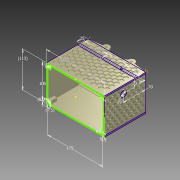
# Autodesk Inventor part: Box2
Saved by Autodesk Inventor 2015 (Build 190159000, 159)
## iProperties
Created: 2015-04-29
Part Number: Box2
Material: Nylon 6/6
Document SubType Name: Modeling
Designer: Akovo_000
Mass: 174.849 g
Surface Area: 2151.16 cm^2
Volume: 154.734 cm^3
Density: 1.13 g/cm^3
Appearance: Nylon 6
Author: Akovo_000
Autodesk Inventor part; units mm, degrees
(part 1 of 2)
ref_plane "YZ Plane" through (0, 0, 0) normal (1, 0, 0) x (0, 1, 0)
ref_plane "XZ Plane" through (0, 0, 0) normal (0, 1, 0) x (-1, 0, 0)
ref_plane "XY Plane" through (0, 0, 0) normal (0, 0, 1) x (1, 0, 0)
sketch "BasicBox" plane through (0, 0, 0) normal (0, 1, 0) x (-1, 0, 0)
  line L0 (88.196, 44.8878) -> (-86.804, 44.8878)
  line L1 (-86.804, 44.8878) -> (-86.804, -60.1122)
  line L2 (-86.804, -60.1122) -> (88.196, -60.1122)
  line L3 (88.196, -60.1122) -> (88.196, 44.8878)
  line L4 (92.196, 48.8878) -> (-90.804, 48.8878)
  line L5 (-90.804, 48.8878) -> (-90.804, -64.1122)
  line L6 (-90.804, -64.1122) -> (92.196, -64.1122)
  line L7 (92.196, -64.1122) -> (92.196, 48.8878)
  line L8 (88.196, 44.8878) -> (88.196, 45.3878) construction
  line L9 (88.196, 44.8878) -> (88.696, 44.8878) construction
  line L10 (88.196, -60.1122) -> (88.196, -60.6122) construction
  line L11 (88.196, -60.1122) -> (88.696, -60.1122) construction
  line L12 (-86.804, -60.1122) -> (-86.804, -60.6122) construction
  line L13 (-86.804, 44.8878) -> (-86.804, 45.3878) construction
  line L14 (-86.804, 44.8878) -> (-87.304, 44.8878) construction
  line L15 (-86.804, -60.1122) -> (-87.304, -60.1122) construction
  line L16 (-87.304, -60.6122) -> (-87.304, -60.1122)
  line L17 (-87.304, 45.3878) -> (-86.804, 45.3878)
  line L18 (88.696, 45.3878) -> (88.696, -60.1122)
  line L19 (88.696, -60.6122) -> (88.196, -60.6122)
  line L20 (88.696, 44.8878) -> (92.196, 44.8878) construction
  line L21 (88.196, 45.3878) -> (88.196, 48.8878) construction
  line L22 (-86.804, 45.3878) -> (88.696, 45.3878)
  line L23 (-87.304, 44.8878) -> (-87.304, 45.3878)
  line L24 (-87.304, -60.1122) -> (-87.304, 44.8878)
  line L25 (-86.804, -60.6122) -> (-87.304, -60.6122)
  line L26 (88.696, -60.1122) -> (88.696, -60.6122)
  line L27 (88.196, -60.6122) -> (-86.804, -60.6122)
  line L28 (88.696, -60.1122) -> (92.196, -60.1122) construction
  line L29 (88.196, -60.6122) -> (88.196, -64.1122) construction
  line L30 (-87.304, 44.8878) -> (-90.804, 44.8878) construction
  line L31 (-86.804, 45.3878) -> (-86.804, 48.8878) construction
  line L32 (-87.304, -60.1122) -> (-90.804, -60.1122) construction
  line L33 (-86.804, -60.6122) -> (-86.804, -64.1122) construction
  line L34 (-76.804, -60.1122) -> (-76.804, -50.1122)
  line L35 (-76.804, -50.1122) -> (-86.804, -50.1122)
  line L36 (-76.804, 44.8878) -> (-76.804, 34.8878)
  line L37 (-76.804, 34.8878) -> (-86.804, 34.8878)
  line L38 (78.696, 44.8878) -> (78.696, 34.8878)
  line L39 (78.696, 34.8878) -> (88.196, 34.8878)
  line L40 (88.696, -50.1122) -> (78.696, -50.1122)
  line L41 (78.696, -50.1122) -> (78.696, -60.1122)
  line L42 (78.696, 44.8878) -> (78.696, 48.8878)
  line L43 (88.196, 34.8878) -> (92.196, 34.8878)
  line L44 (78.696, -60.1122) -> (78.696, -64.1122)
  line L45 (88.696, -50.1122) -> (92.196, -50.1122)
  line L46 (-80.7418, -53.1122) -> (-78.721, -56.6122)
  line L47 (-78.721, -56.6122) -> (-80.7418, -60.1122)
  line L48 (-80.7418, -60.1122) -> (-84.7832, -60.1122)
  line L49 (-84.7832, -60.1122) -> (-86.804, -56.6122)
  line L50 (-86.804, -56.6122) -> (-84.7832, -53.1122)
  line L51 (-84.7832, -53.1122) -> (-80.7418, -53.1122)
  line L52 (-80.7418, 44.8878) -> (-78.721, 41.3878)
  line L53 (-78.721, 41.3878) -> (-80.7418, 37.8878)
  line L54 (-80.7418, 37.8878) -> (-84.7832, 37.8878)
  line L55 (-84.7832, 37.8878) -> (-86.804, 41.3878)
  line L56 (-86.804, 41.3878) -> (-84.7832, 44.8878)
  line L57 (-84.7832, 44.8878) -> (-80.7418, 44.8878)
  line L58 (86.1753, 44.8878) -> (88.196, 41.3878)
  line L59 (88.196, 41.3878) -> (86.1753, 37.8878)
  line L60 (86.1753, 37.8878) -> (82.1339, 37.8878)
  line L61 (82.1339, 37.8878) -> (80.1131, 41.3878)
  line L62 (80.1131, 41.3878) -> (82.1339, 44.8878)
  line L63 (82.1339, 44.8878) -> (86.1753, 44.8878)
  line L64 (86.1753, -53.1122) -> (88.196, -56.6122)
  line L65 (88.196, -56.6122) -> (86.1753, -60.1122)
  line L66 (86.1753, -60.1122) -> (82.1339, -60.1122)
  line L67 (82.1339, -60.1122) -> (80.1131, -56.6122)
  line L68 (80.1131, -56.6122) -> (82.1339, -53.1122)
  line L69 (82.1339, -53.1122) -> (86.1753, -53.1122)
  circle A0 centre (84.1546, 41.3878) radius 2
  circle A1 centre (84.1546, -56.6122) radius 2
  circle A2 centre (-82.7625, -56.6122) radius 2
  circle A3 centre (-82.7625, 41.3878) radius 2
  point P0 (0, 0)
  dimension "d2" = 105
  dimension "d3" = 175
  dimension "d4" = 4
  dimension "d68" = 0.5
  dimension "d71" = 4
  dimension "d94" = 10
  dimension "d95" = 183
  dimension "d96" = 113
  dimension "d97" = 7
  dimension "d98" = 0
  dimension "d101" = 0
  dimension "d102" = 4
  dimension "d105" = 0
  dimension "d106" = 0
  dimension "d109" = 7.5
  dimension "d110" = 8.0414
  constraints: 140 end point, 29 point on line, 22 perpendicular, 14 equal length, 9 parallel, 6 vertical, 5 collinear, 4 centre point, 4 coincident, 4 horizontal, 3 equal radius, 52 other
  measures "d2" distance of L28.end L20.end
  measures "d3" distance of L29.end L33.end
  measures "d4" distance of L6.end L28.end
  measures "d68" distance of L16.start L12.end
  measures "d71" distance of L6.end L29.end
  measures "d94" distance of L34.start L34.end
  measures "d95" distance between parallel lines of L7 L5
  measures "d96" distance between parallel lines of L4 L6
  measures "d97" distance between parallel lines of L51 L48
  measures "d98" distance from line of L1 L49.end
  measures "d101" distance from line of L3 L64.end
  measures "d102" diameter of A0
  measures "d105" distance from line of L1 L55.end
  measures "d106" distance from line of L3 L58.end
  measures "d109" distance from line of L6 point (84.155, -56.612)
  measures "d110" distance from line of L7 point (84.155, -56.612)
extrude "Extrusion1" add sketch "BasicBox" along normal blind 131 contours L0 L42 L22 L18 L43 L3 | L43 L18 L40 L3 | L0 L1 L2 L44 L27 L25 L16 L24 L23 L17 L22 L42 | L40 L18 L26 L19 L27 L44 L2 L3 | L43 L7 L45 L18 | L18 L22 L42 L4 L7 L43 | L22 L17 L23 L24 L16 L25 L27 L44 L6 L5 L4 L42 | L45 L7 L6 L44 L27 L19 L26 L18
sketch "LongerHonycomb" plane through (-92.196, 0, 48.8878) normal (0, 0, 1) x (1, 0, 0)
  line L0 (0, 131) -> (183, 131)
  line L1 (183, 131) -> (183, 0)
  line L2 (183, 0) -> (0, 0)
  line L3 (0, 0) -> (0, 131)
  line L4 (0, 131) -> (183, 131) projected
  line L5 (179, 131) -> (179, 0)
  line L6 (4, 131) -> (4, 0)
  line L7 (179, 131) -> (4, 131) projected
  line L8 (4, 0) -> (179, 0) projected
  line L9 (18.2583, 115) -> (10.7528, 115)
  line L10 (10.7528, 115) -> (7, 121.5)
  line L11 (7, 121.5) -> (10.7528, 128)
  line L12 (10.7528, 128) -> (18.2583, 128)
  line L13 (18.2583, 128) -> (22.0111, 121.5)
  line L14 (22.0111, 121.5) -> (18.2583, 115)
  line L15 (33.8468, 114) -> (30.094, 107.5)
  line L16 (30.094, 107.5) -> (22.5885, 107.5)
  line L17 (22.5885, 107.5) -> (18.8357, 114)
  line L18 (18.8357, 114) -> (22.5885, 120.5)
  line L19 (22.5885, 120.5) -> (30.094, 120.5)
  line L20 (30.094, 120.5) -> (33.8468, 114)
  line L21 (41.9583, 115) -> (34.4528, 115)
  line L22 (34.4528, 115) -> (30.7, 121.5)
  line L23 (30.7, 121.5) -> (34.4528, 128)
  line L24 (34.4528, 128) -> (41.9583, 128)
  line L25 (41.9583, 128) -> (45.7111, 121.5)
  line L26 (45.7111, 121.5) -> (41.9583, 115)
  line L27 (57.5468, 114) -> (53.794, 107.5)
  line L28 (53.794, 107.5) -> (46.2885, 107.5)
  line L29 (46.2885, 107.5) -> (42.5357, 114)
  line L30 (42.5357, 114) -> (46.2885, 120.5)
  line L31 (46.2885, 120.5) -> (53.794, 120.5)
  line L32 (53.794, 120.5) -> (57.5468, 114)
  line L33 (65.6583, 115) -> (58.1528, 115)
  line L34 (58.1528, 115) -> (54.4, 121.5)
  line L35 (54.4, 121.5) -> (58.1528, 128)
  line L36 (58.1528, 128) -> (65.6583, 128)
  line L37 (65.6583, 128) -> (69.4111, 121.5)
  line L38 (69.4111, 121.5) -> (65.6583, 115)
  line L39 (81.2468, 114) -> (77.494, 107.5)
  line L40 (77.494, 107.5) -> (69.9885, 107.5)
  line L41 (69.9885, 107.5) -> (66.2357, 114)
  line L42 (66.2357, 114) -> (69.9885, 120.5)
  line L43 (69.9885, 120.5) -> (77.494, 120.5)
  line L44 (77.494, 120.5) -> (81.2468, 114)
  line L45 (89.3583, 115) -> (81.8528, 115)
  line L46 (81.8528, 115) -> (78.1, 121.5)
  line L47 (78.1, 121.5) -> (81.8528, 128)
  line L48 (81.8528, 128) -> (89.3583, 128)
  line L49 (89.3583, 128) -> (93.1111, 121.5)
  line L50 (93.1111, 121.5) -> (89.3583, 115)
  line L51 (104.9468, 114) -> (101.194, 107.5)
  line L52 (101.194, 107.5) -> (93.6885, 107.5)
  line L53 (93.6885, 107.5) -> (89.9357, 114)
  line L54 (89.9357, 114) -> (93.6885, 120.5)
  line L55 (93.6885, 120.5) -> (101.194, 120.5)
  line L56 (101.194, 120.5) -> (104.9468, 114)
  line L57 (113.0583, 115) -> (105.5528, 115)
  line L58 (105.5528, 115) -> (101.8, 121.5)
  line L59 (101.8, 121.5) -> (105.5528, 128)
  line L60 (105.5528, 128) -> (113.0583, 128)
  line L61 (113.0583, 128) -> (116.8111, 121.5)
  line L62 (116.8111, 121.5) -> (113.0583, 115)
  line L63 (128.6468, 114) -> (124.894, 107.5)
  line L64 (124.894, 107.5) -> (117.3885, 107.5)
  line L65 (117.3885, 107.5) -> (113.6357, 114)
  line L66 (113.6357, 114) -> (117.3885, 120.5)
  line L67 (117.3885, 120.5) -> (124.894, 120.5)
  line L68 (124.894, 120.5) -> (128.6468, 114)
  line L69 (136.7583, 115) -> (129.2528, 115)
  line L70 (129.2528, 115) -> (125.5, 121.5)
  line L71 (125.5, 121.5) -> (129.2528, 128)
  line L72 (129.2528, 128) -> (136.7583, 128)
  line L73 (136.7583, 128) -> (140.5111, 121.5)
  line L74 (140.5111, 121.5) -> (136.7583, 115)
  line L75 (152.3468, 114) -> (148.594, 107.5)
  line L76 (148.594, 107.5) -> (141.0885, 107.5)
  line L77 (141.0885, 107.5) -> (137.3357, 114)
  line L78 (137.3357, 114) -> (141.0885, 120.5)
  line L79 (141.0885, 120.5) -> (148.594, 120.5)
  line L80 (148.594, 120.5) -> (152.3468, 114)
  line L81 (18.2583, 100) -> (10.7528, 100)
  line L82 (10.7528, 100) -> (7, 106.5)
  line L83 (7, 106.5) -> (10.7528, 113)
  line L84 (10.7528, 113) -> (18.2583, 113)
  line L85 (18.2583, 113) -> (22.0111, 106.5)
  line L86 (22.0111, 106.5) -> (18.2583, 100)
  line L87 (33.8468, 99) -> (30.094, 92.5)
  line L88 (30.094, 92.5) -> (22.5885, 92.5)
  line L89 (22.5885, 92.5) -> (18.8357, 99)
  line L90 (18.8357, 99) -> (22.5885, 105.5)
  line L91 (22.5885, 105.5) -> (30.094, 105.5)
  line L92 (30.094, 105.5) -> (33.8468, 99)
  line L93 (41.9583, 100) -> (34.4528, 100)
  line L94 (34.4528, 100) -> (30.7, 106.5)
  line L95 (30.7, 106.5) -> (34.4528, 113)
  line L96 (34.4528, 113) -> (41.9583, 113)
  line L97 (41.9583, 113) -> (45.7111, 106.5)
  line L98 (45.7111, 106.5) -> (41.9583, 100)
  line L99 (57.5468, 99) -> (53.794, 92.5)
  line L100 (53.794, 92.5) -> (46.2885, 92.5)
  line L101 (46.2885, 92.5) -> (42.5357, 99)
  line L102 (42.5357, 99) -> (46.2885, 105.5)
  line L103 (46.2885, 105.5) -> (53.794, 105.5)
  line L104 (53.794, 105.5) -> (57.5468, 99)
  line L105 (65.6583, 100) -> (58.1528, 100)
  line L106 (58.1528, 100) -> (54.4, 106.5)
  line L107 (54.4, 106.5) -> (58.1528, 113)
  line L108 (58.1528, 113) -> (65.6583, 113)
  line L109 (65.6583, 113) -> (69.4111, 106.5)
  line L110 (69.4111, 106.5) -> (65.6583, 100)
  line L111 (81.2468, 99) -> (77.494, 92.5)
  line L112 (77.494, 92.5) -> (69.9885, 92.5)
  line L113 (69.9885, 92.5) -> (66.2357, 99)
  line L114 (66.2357, 99) -> (69.9885, 105.5)
  line L115 (69.9885, 105.5) -> (77.494, 105.5)
  line L116 (77.494, 105.5) -> (81.2468, 99)
  line L117 (89.3583, 100) -> (81.8528, 100)
  line L118 (81.8528, 100) -> (78.1, 106.5)
  line L119 (78.1, 106.5) -> (81.8528, 113)
  line L120 (81.8528, 113) -> (89.3583, 113)
  line L121 (89.3583, 113) -> (93.1111, 106.5)
  line L122 (93.1111, 106.5) -> (89.3583, 100)
  line L123 (104.9468, 99) -> (101.194, 92.5)
  line L124 (101.194, 92.5) -> (93.6885, 92.5)
  line L125 (93.6885, 92.5) -> (89.9357, 99)
  line L126 (89.9357, 99) -> (93.6885, 105.5)
  line L127 (93.6885, 105.5) -> (101.194, 105.5)
  line L128 (101.194, 105.5) -> (104.9468, 99)
  line L129 (113.0583, 100) -> (105.5528, 100)
  line L130 (105.5528, 100) -> (101.8, 106.5)
  line L131 (101.8, 106.5) -> (105.5528, 113)
  line L132 (105.5528, 113) -> (113.0583, 113)
  line L133 (113.0583, 113) -> (116.8111, 106.5)
  line L134 (116.8111, 106.5) -> (113.0583, 100)
  line L135 (128.6468, 99) -> (124.894, 92.5)
  line L136 (124.894, 92.5) -> (117.3885, 92.5)
  line L137 (117.3885, 92.5) -> (113.6357, 99)
  line L138 (113.6357, 99) -> (117.3885, 105.5)
  line L139 (117.3885, 105.5) -> (124.894, 105.5)
  line L140 (124.894, 105.5) -> (128.6468, 99)
  line L141 (136.7583, 100) -> (129.2528, 100)
  line L142 (129.2528, 100) -> (125.5, 106.5)
  line L143 (125.5, 106.5) -> (129.2528, 113)
  line L144 (129.2528, 113) -> (136.7583, 113)
  line L145 (136.7583, 113) -> (140.5111, 106.5)
  line L146 (140.5111, 106.5) -> (136.7583, 100)
  line L147 (152.3468, 99) -> (148.594, 92.5)
  line L148 (148.594, 92.5) -> (141.0885, 92.5)
  line L149 (141.0885, 92.5) -> (137.3357, 99)
  line L150 (137.3357, 99) -> (141.0885, 105.5)
  line L151 (141.0885, 105.5) -> (148.594, 105.5)
  line L152 (148.594, 105.5) -> (152.3468, 99)
  line L153 (18.2583, 85) -> (10.7528, 85)
  line L154 (10.7528, 85) -> (7, 91.5)
  line L155 (7, 91.5) -> (10.7528, 98)
  line L156 (10.7528, 98) -> (18.2583, 98)
  line L157 (18.2583, 98) -> (22.0111, 91.5)
  line L158 (22.0111, 91.5) -> (18.2583, 85)
  line L159 (33.8468, 84) -> (30.094, 77.5)
  line L160 (30.094, 77.5) -> (22.5885, 77.5)
  line L161 (22.5885, 77.5) -> (18.8357, 84)
  line L162 (18.8357, 84) -> (22.5885, 90.5)
  line L163 (22.5885, 90.5) -> (30.094, 90.5)
  line L164 (30.094, 90.5) -> (33.8468, 84)
  line L165 (41.9583, 85) -> (34.4528, 85)
  line L166 (34.4528, 85) -> (30.7, 91.5)
  line L167 (30.7, 91.5) -> (34.4528, 98)
  line L168 (34.4528, 98) -> (41.9583, 98)
  line L169 (41.9583, 98) -> (45.7111, 91.5)
  line L170 (45.7111, 91.5) -> (41.9583, 85)
  line L171 (57.5468, 84) -> (53.794, 77.5)
  line L172 (53.794, 77.5) -> (46.2885, 77.5)
  line L173 (46.2885, 77.5) -> (42.5357, 84)
  line L174 (42.5357, 84) -> (46.2885, 90.5)
  line L175 (46.2885, 90.5) -> (53.794, 90.5)
  line L176 (53.794, 90.5) -> (57.5468, 84)
  line L177 (65.6583, 85) -> (58.1528, 85)
  line L178 (58.1528, 85) -> (54.4, 91.5)
  line L179 (54.4, 91.5) -> (58.1528, 98)
  line L180 (58.1528, 98) -> (65.6583, 98)
  line L181 (65.6583, 98) -> (69.4111, 91.5)
  line L182 (69.4111, 91.5) -> (65.6583, 85)
  line L183 (81.2468, 84) -> (77.494, 77.5)
  line L184 (77.494, 77.5) -> (69.9885, 77.5)
  line L185 (69.9885, 77.5) -> (66.2357, 84)
  line L186 (66.2357, 84) -> (69.9885, 90.5)
  line L187 (69.9885, 90.5) -> (77.494, 90.5)
  line L188 (77.494, 90.5) -> (81.2468, 84)
  line L189 (89.3583, 85) -> (81.8528, 85)
  line L190 (81.8528, 85) -> (78.1, 91.5)
  line L191 (78.1, 91.5) -> (81.8528, 98)
  line L192 (81.8528, 98) -> (89.3583, 98)
  line L193 (89.3583, 98) -> (93.1111, 91.5)
  line L194 (93.1111, 91.5) -> (89.3583, 85)
  line L195 (104.9468, 84) -> (101.194, 77.5)
  line L196 (101.194, 77.5) -> (93.6885, 77.5)
  line L197 (93.6885, 77.5) -> (89.9357, 84)
  line L198 (89.9357, 84) -> (93.6885, 90.5)
  line L199 (93.6885, 90.5) -> (101.194, 90.5)
  line L200 (101.194, 90.5) -> (104.9468, 84)
  line L201 (113.0583, 85) -> (105.5528, 85)
  line L202 (105.5528, 85) -> (101.8, 91.5)
  line L203 (101.8, 91.5) -> (105.5528, 98)
  line L204 (105.5528, 98) -> (113.0583, 98)
  line L205 (113.0583, 98) -> (116.8111, 91.5)
  line L206 (116.8111, 91.5) -> (113.0583, 85)
  line L207 (128.6468, 84) -> (124.894, 77.5)
  line L208 (124.894, 77.5) -> (117.3885, 77.5)
  line L209 (117.3885, 77.5) -> (113.6357, 84)
  line L210 (113.6357, 84) -> (117.3885, 90.5)
  line L211 (117.3885, 90.5) -> (124.894, 90.5)
  line L212 (124.894, 90.5) -> (128.6468, 84)
  line L213 (136.7583, 85) -> (129.2528, 85)
  line L214 (129.2528, 85) -> (125.5, 91.5)
  line L215 (125.5, 91.5) -> (129.2528, 98)
  line L216 (129.2528, 98) -> (136.7583, 98)
  line L217 (136.7583, 98) -> (140.5111, 91.5)
  line L218 (140.5111, 91.5) -> (136.7583, 85)
  line L219 (152.3468, 84) -> (148.594, 77.5)
  line L220 (148.594, 77.5) -> (141.0885, 77.5)
  line L221 (141.0885, 77.5) -> (137.3357, 84)
  line L222 (137.3357, 84) -> (141.0885, 90.5)
  line L223 (141.0885, 90.5) -> (148.594, 90.5)
  line L224 (148.594, 90.5) -> (152.3468, 84)
  line L225 (18.2583, 70) -> (10.7528, 70)
  line L226 (10.7528, 70) -> (7, 76.5)
  line L227 (7, 76.5) -> (10.7528, 83)
  line L228 (10.7528, 83) -> (18.2583, 83)
  line L229 (18.2583, 83) -> (22.0111, 76.5)
  line L230 (22.0111, 76.5) -> (18.2583, 70)
  line L231 (33.8468, 69) -> (30.094, 62.5)
  line L232 (30.094, 62.5) -> (22.5885, 62.5)
  line L233 (22.5885, 62.5) -> (18.8357, 69)
  line L234 (18.8357, 69) -> (22.5885, 75.5)
  line L235 (22.5885, 75.5) -> (30.094, 75.5)
  line L236 (30.094, 75.5) -> (33.8468, 69)
  line L237 (41.9583, 70) -> (34.4528, 70)
  line L238 (34.4528, 70) -> (30.7, 76.5)
  line L239 (30.7, 76.5) -> (34.4528, 83)
  line L240 (34.4528, 83) -> (41.9583, 83)
  line L241 (41.9583, 83) -> (45.7111, 76.5)
  line L242 (45.7111, 76.5) -> (41.9583, 70)
  line L243 (57.5468, 69) -> (53.794, 62.5)
  line L244 (53.794, 62.5) -> (46.2885, 62.5)
  line L245 (46.2885, 62.5) -> (42.5357, 69)
  line L246 (42.5357, 69) -> (46.2885, 75.5)
  line L247 (46.2885, 75.5) -> (53.794, 75.5)
  line L248 (53.794, 75.5) -> (57.5468, 69)
  line L249 (65.6583, 70) -> (58.1528, 70)
  line L250 (58.1528, 70) -> (54.4, 76.5)
  line L251 (54.4, 76.5) -> (58.1528, 83)
  line L252 (58.1528, 83) -> (65.6583, 83)
  line L253 (65.6583, 83) -> (69.4111, 76.5)
  line L254 (69.4111, 76.5) -> (65.6583, 70)
  line L255 (81.2468, 69) -> (77.494, 62.5)
  line L256 (77.494, 62.5) -> (69.9885, 62.5)
  line L257 (69.9885, 62.5) -> (66.2357, 69)
  line L258 (66.2357, 69) -> (69.9885, 75.5)
  line L259 (69.9885, 75.5) -> (77.494, 75.5)
  line L260 (77.494, 75.5) -> (81.2468, 69)
  line L261 (89.3583, 70) -> (81.8528, 70)
  line L262 (81.8528, 70) -> (78.1, 76.5)
  line L263 (78.1, 76.5) -> (81.8528, 83)
  line L264 (81.8528, 83) -> (89.3583, 83)
  line L265 (89.3583, 83) -> (93.1111, 76.5)
  line L266 (93.1111, 76.5) -> (89.3583, 70)
  line L267 (104.9468, 69) -> (101.194, 62.5)
  line L268 (101.194, 62.5) -> (93.6885, 62.5)
  line L269 (93.6885, 62.5) -> (89.9357, 69)
  line L270 (89.9357, 69) -> (93.6885, 75.5)
  line L271 (93.6885, 75.5) -> (101.194, 75.5)
  line L272 (101.194, 75.5) -> (104.9468, 69)
  line L273 (113.0583, 70) -> (105.5528, 70)
  line L274 (105.5528, 70) -> (101.8, 76.5)
  line L275 (101.8, 76.5) -> (105.5528, 83)
  line L276 (105.5528, 83) -> (113.0583, 83)
  line L277 (113.0583, 83) -> (116.8111, 76.5)
  line L278 (116.8111, 76.5) -> (113.0583, 70)
  line L279 (128.6468, 69) -> (124.894, 62.5)
  line L280 (124.894, 62.5) -> (117.3885, 62.5)
  line L281 (117.3885, 62.5) -> (113.6357, 69)
  line L282 (113.6357, 69) -> (117.3885, 75.5)
  line L283 (117.3885, 75.5) -> (124.894, 75.5)
  line L284 (124.894, 75.5) -> (128.6468, 69)
  line L285 (136.7583, 70) -> (129.2528, 70)
  line L286 (129.2528, 70) -> (125.5, 76.5)
  line L287 (125.5, 76.5) -> (129.2528, 83)
  line L288 (129.2528, 83) -> (136.7583, 83)
  line L289 (136.7583, 83) -> (140.5111, 76.5)
  line L290 (140.5111, 76.5) -> (136.7583, 70)
  line L291 (152.3468, 69) -> (148.594, 62.5)
  line L292 (148.594, 62.5) -> (141.0885, 62.5)
  line L293 (141.0885, 62.5) -> (137.3357, 69)
  line L294 (137.3357, 69) -> (141.0885, 75.5)
  line L295 (141.0885, 75.5) -> (148.594, 75.5)
  line L296 (148.594, 75.5) -> (152.3468, 69)
  line L297 (18.2583, 55) -> (10.7528, 55)
  line L298 (10.7528, 55) -> (7, 61.5)
  line L299 (7, 61.5) -> (10.7528, 68)
  line L300 (10.7528, 68) -> (18.2583, 68)
  line L301 (18.2583, 68) -> (22.0111, 61.5)
  line L302 (22.0111, 61.5) -> (18.2583, 55)
  line L303 (33.8468, 54) -> (30.094, 47.5)
  line L304 (30.094, 47.5) -> (22.5885, 47.5)
  line L305 (22.5885, 47.5) -> (18.8357, 54)
  line L306 (18.8357, 54) -> (22.5885, 60.5)
  line L307 (22.5885, 60.5) -> (30.094, 60.5)
  line L308 (30.094, 60.5) -> (33.8468, 54)
  line L309 (41.9583, 55) -> (34.4528, 55)
  line L310 (34.4528, 55) -> (30.7, 61.5)
  line L311 (30.7, 61.5) -> (34.4528, 68)
  line L312 (34.4528, 68) -> (41.9583, 68)
  line L313 (41.9583, 68) -> (45.7111, 61.5)
  line L314 (45.7111, 61.5) -> (41.9583, 55)
  line L315 (57.5468, 54) -> (53.794, 47.5)
  line L316 (53.794, 47.5) -> (46.2885, 47.5)
  line L317 (46.2885, 47.5) -> (42.5357, 54)
  line L318 (42.5357, 54) -> (46.2885, 60.5)
  line L319 (46.2885, 60.5) -> (53.794, 60.5)
  line L320 (53.794, 60.5) -> (57.5468, 54)
  line L321 (65.6583, 55) -> (58.1528, 55)
  line L322 (58.1528, 55) -> (54.4, 61.5)
  line L323 (54.4, 61.5) -> (58.1528, 68)
  line L324 (58.1528, 68) -> (65.6583, 68)
  line L325 (65.6583, 68) -> (69.4111, 61.5)
  line L326 (69.4111, 61.5) -> (65.6583, 55)
  line L327 (81.2468, 54) -> (77.494, 47.5)
  line L328 (77.494, 47.5) -> (69.9885, 47.5)
  line L329 (69.9885, 47.5) -> (66.2357, 54)
  line L330 (66.2357, 54) -> (69.9885, 60.5)
  line L331 (69.9885, 60.5) -> (77.494, 60.5)
  line L332 (77.494, 60.5) -> (81.2468, 54)
  line L333 (89.3583, 55) -> (81.8528, 55)
  line L334 (81.8528, 55) -> (78.1, 61.5)
  line L335 (78.1, 61.5) -> (81.8528, 68)
  line L336 (81.8528, 68) -> (89.3583, 68)
  line L337 (89.3583, 68) -> (93.1111, 61.5)
  line L338 (93.1111, 61.5) -> (89.3583, 55)
  line L339 (104.9468, 54) -> (101.194, 47.5)
  line L340 (101.194, 47.5) -> (93.6885, 47.5)
  line L341 (93.6885, 47.5) -> (89.9357, 54)
  line L342 (89.9357, 54) -> (93.6885, 60.5)
  line L343 (93.6885, 60.5) -> (101.194, 60.5)
  line L344 (101.194, 60.5) -> (104.9468, 54)
  line L345 (113.0583, 55) -> (105.5528, 55)
  line L346 (105.5528, 55) -> (101.8, 61.5)
  line L347 (101.8, 61.5) -> (105.5528, 68)
  line L348 (105.5528, 68) -> (113.0583, 68)
  line L349 (113.0583, 68) -> (116.8111, 61.5)
  line L350 (116.8111, 61.5) -> (113.0583, 55)
  line L351 (128.6468, 54) -> (124.894, 47.5)
  line L352 (124.894, 47.5) -> (117.3885, 47.5)
  line L353 (117.3885, 47.5) -> (113.6357, 54)
  line L354 (113.6357, 54) -> (117.3885, 60.5)
  line L355 (117.3885, 60.5) -> (124.894, 60.5)
  line L356 (124.894, 60.5) -> (128.6468, 54)
  line L357 (136.7583, 55) -> (129.2528, 55)
  line L358 (129.2528, 55) -> (125.5, 61.5)
  line L359 (125.5, 61.5) -> (129.2528, 68)
  line L360 (129.2528, 68) -> (136.7583, 68)
  line L361 (136.7583, 68) -> (140.5111, 61.5)
  line L362 (140.5111, 61.5) -> (136.7583, 55)
  line L363 (152.3468, 54) -> (148.594, 47.5)
  line L364 (148.594, 47.5) -> (141.0885, 47.5)
  line L365 (141.0885, 47.5) -> (137.3357, 54)
  line L366 (137.3357, 54) -> (141.0885, 60.5)
  line L367 (141.0885, 60.5) -> (148.594, 60.5)
  line L368 (148.594, 60.5) -> (152.3468, 54)
  line L369 (18.2583, 40) -> (10.7528, 40)
  line L370 (10.7528, 40) -> (7, 46.5)
  line L371 (7, 46.5) -> (10.7528, 53)
  line L372 (10.7528, 53) -> (18.2583, 53)
  line L373 (18.2583, 53) -> (22.0111, 46.5)
  line L374 (22.0111, 46.5) -> (18.2583, 40)
  line L375 (33.8468, 39) -> (30.094, 32.5)
  line L376 (30.094, 32.5) -> (22.5885, 32.5)
  line L377 (22.5885, 32.5) -> (18.8357, 39)
  line L378 (18.8357, 39) -> (22.5885, 45.5)
  line L379 (22.5885, 45.5) -> (30.094, 45.5)
  line L380 (30.094, 45.5) -> (33.8468, 39)
  line L381 (41.9583, 40) -> (34.4528, 40)
  line L382 (34.4528, 40) -> (30.7, 46.5)
  line L383 (30.7, 46.5) -> (34.4528, 53)
  line L384 (34.4528, 53) -> (41.9583, 53)
  line L385 (41.9583, 53) -> (45.7111, 46.5)
  line L386 (45.7111, 46.5) -> (41.9583, 40)
  line L387 (57.5468, 39) -> (53.794, 32.5)
  line L388 (53.794, 32.5) -> (46.2885, 32.5)
  line L389 (46.2885, 32.5) -> (42.5357, 39)
  line L390 (42.5357, 39) -> (46.2885, 45.5)
  line L391 (46.2885, 45.5) -> (53.794, 45.5)
  line L392 (53.794, 45.5) -> (57.5468, 39)
  line L393 (65.6583, 40) -> (58.1528, 40)
  line L394 (58.1528, 40) -> (54.4, 46.5)
  line L395 (54.4, 46.5) -> (58.1528, 53)
  line L396 (58.1528, 53) -> (65.6583, 53)
  line L397 (65.6583, 53) -> (69.4111, 46.5)
  line L398 (69.4111, 46.5) -> (65.6583, 40)
  line L399 (81.2468, 39) -> (77.494, 32.5)
  line L400 (77.494, 32.5) -> (69.9885, 32.5)
  line L401 (69.9885, 32.5) -> (66.2357, 39)
  line L402 (66.2357, 39) -> (69.9885, 45.5)
  line L403 (69.9885, 45.5) -> (77.494, 45.5)
  line L404 (77.494, 45.5) -> (81.2468, 39)
  line L405 (89.3583, 40) -> (81.8528, 40)
  line L406 (81.8528, 40) -> (78.1, 46.5)
  line L407 (78.1, 46.5) -> (81.8528, 53)
  line L408 (81.8528, 53) -> (89.3583, 53)
  line L409 (89.3583, 53) -> (93.1111, 46.5)
  line L410 (93.1111, 46.5) -> (89.3583, 40)
  line L411 (104.9468, 39) -> (101.194, 32.5)
  line L412 (101.194, 32.5) -> (93.6885, 32.5)
  line L413 (93.6885, 32.5) -> (89.9357, 39)
  line L414 (89.9357, 39) -> (93.6885, 45.5)
  line L415 (93.6885, 45.5) -> (101.194, 45.5)
  line L416 (101.194, 45.5) -> (104.9468, 39)
  line L417 (113.0583, 40) -> (105.5528, 40)
  line L418 (105.5528, 40) -> (101.8, 46.5)
  line L419 (101.8, 46.5) -> (105.5528, 53)
  line L420 (105.5528, 53) -> (113.0583, 53)
  line L421 (113.0583, 53) -> (116.8111, 46.5)
  line L422 (116.8111, 46.5) -> (113.0583, 40)
  line L423 (128.6468, 39) -> (124.894, 32.5)
  line L424 (124.894, 32.5) -> (117.3885, 32.5)
  line L425 (117.3885, 32.5) -> (113.6357, 39)
  line L426 (113.6357, 39) -> (117.3885, 45.5)
  line L427 (117.3885, 45.5) -> (124.894, 45.5)
  line L428 (124.894, 45.5) -> (128.6468, 39)
  line L429 (136.7583, 40) -> (129.2528, 40)
  line L430 (129.2528, 40) -> (125.5, 46.5)
  line L431 (125.5, 46.5) -> (129.2528, 53)
  line L432 (129.2528, 53) -> (136.7583, 53)
  line L433 (136.7583, 53) -> (140.5111, 46.5)
  line L434 (140.5111, 46.5) -> (136.7583, 40)
  line L435 (152.3468, 39) -> (148.594, 32.5)
  line L436 (148.594, 32.5) -> (141.0885, 32.5)
  line L437 (141.0885, 32.5) -> (137.3357, 39)
  line L438 (137.3357, 39) -> (141.0885, 45.5)
  line L439 (141.0885, 45.5) -> (148.594, 45.5)
  line L440 (148.594, 45.5) -> (152.3468, 39)
  line L441 (18.2583, 25) -> (10.7528, 25)
  line L442 (10.7528, 25) -> (7, 31.5)
  line L443 (7, 31.5) -> (10.7528, 38)
  line L444 (10.7528, 38) -> (18.2583, 38)
  line L445 (18.2583, 38) -> (22.0111, 31.5)
  line L446 (22.0111, 31.5) -> (18.2583, 25)
  line L447 (33.8468, 24) -> (30.094, 17.5)
  line L448 (30.094, 17.5) -> (22.5885, 17.5)
  line L449 (22.5885, 17.5) -> (18.8357, 24)
  line L450 (18.8357, 24) -> (22.5885, 30.5)
  line L451 (22.5885, 30.5) -> (30.094, 30.5)
  line L452 (30.094, 30.5) -> (33.8468, 24)
  line L453 (41.9583, 25) -> (34.4528, 25)
  line L454 (34.4528, 25) -> (30.7, 31.5)
  line L455 (30.7, 31.5) -> (34.4528, 38)
  line L456 (34.4528, 38) -> (41.9583, 38)
  line L457 (41.9583, 38) -> (45.7111, 31.5)
  line L458 (45.7111, 31.5) -> (41.9583, 25)
  line L459 (57.5468, 24) -> (53.794, 17.5)
  line L460 (53.794, 17.5) -> (46.2885, 17.5)
  line L461 (46.2885, 17.5) -> (42.5357, 24)
  line L462 (42.5357, 24) -> (46.2885, 30.5)
  line L463 (46.2885, 30.5) -> (53.794, 30.5)
  line L464 (53.794, 30.5) -> (57.5468, 24)
  line L465 (65.6583, 25) -> (58.1528, 25)
  line L466 (58.1528, 25) -> (54.4, 31.5)
  line L467 (54.4, 31.5) -> (58.1528, 38)
  line L468 (58.1528, 38) -> (65.6583, 38)
  line L469 (65.6583, 38) -> (69.4111, 31.5)
  line L470 (69.4111, 31.5) -> (65.6583, 25)
  line L471 (81.2468, 24) -> (77.494, 17.5)
  line L472 (77.494, 17.5) -> (69.9885, 17.5)
  line L473 (69.9885, 17.5) -> (66.2357, 24)
  line L474 (66.2357, 24) -> (69.9885, 30.5)
  line L475 (69.9885, 30.5) -> (77.494, 30.5)
  line L476 (77.494, 30.5) -> (81.2468, 24)
  line L477 (89.3583, 25) -> (81.8528, 25)
  line L478 (81.8528, 25) -> (78.1, 31.5)
  line L479 (78.1, 31.5) -> (81.8528, 38)
  line L480 (81.8528, 38) -> (89.3583, 38)
  line L481 (89.3583, 38) -> (93.1111, 31.5)
  line L482 (93.1111, 31.5) -> (89.3583, 25)
  line L483 (104.9468, 24) -> (101.194, 17.5)
  line L484 (101.194, 17.5) -> (93.6885, 17.5)
  line L485 (93.6885, 17.5) -> (89.9357, 24)
  line L486 (89.9357, 24) -> (93.6885, 30.5)
  line L487 (93.6885, 30.5) -> (101.194, 30.5)
  line L488 (101.194, 30.5) -> (104.9468, 24)
  line L489 (113.0583, 25) -> (105.5528, 25)
  line L490 (105.5528, 25) -> (101.8, 31.5)
  line L491 (101.8, 31.5) -> (105.5528, 38)
  line L492 (105.5528, 38) -> (113.0583, 38)
  line L493 (113.0583, 38) -> (116.8111, 31.5)
  line L494 (116.8111, 31.5) -> (113.0583, 25)
  line L495 (128.6468, 24) -> (124.894, 17.5)
  line L496 (124.894, 17.5) -> (117.3885, 17.5)
  line L497 (117.3885, 17.5) -> (113.6357, 24)
  line L498 (113.6357, 24) -> (117.3885, 30.5)
  line L499 (117.3885, 30.5) -> (124.894, 30.5)
  line L500 (124.894, 30.5) -> (128.6468, 24)
  line L501 (136.7583, 25) -> (129.2528, 25)
  line L502 (129.2528, 25) -> (125.5, 31.5)
  line L503 (125.5, 31.5) -> (129.2528, 38)
  line L504 (129.2528, 38) -> (136.7583, 38)
  line L505 (136.7583, 38) -> (140.5111, 31.5)
  line L506 (140.5111, 31.5) -> (136.7583, 25)
  line L507 (152.3468, 24) -> (148.594, 17.5)
  line L508 (148.594, 17.5) -> (141.0885, 17.5)
  line L509 (141.0885, 17.5) -> (137.3357, 24)
  line L510 (137.3357, 24) -> (141.0885, 30.5)
  line L511 (141.0885, 30.5) -> (148.594, 30.5)
  line L512 (148.594, 30.5) -> (152.3468, 24)
  line L513 (18.2583, 10) -> (10.7528, 10)
  line L514 (10.7528, 10) -> (7, 16.5)
  line L515 (7, 16.5) -> (10.7528, 23)
  line L516 (10.7528, 23) -> (18.2583, 23)
  line L517 (18.2583, 23) -> (22.0111, 16.5)
  line L518 (22.0111, 16.5) -> (18.2583, 10)
  line L519 (41.9583, 10) -> (34.4528, 10)
  line L520 (34.4528, 10) -> (30.7, 16.5)
  line L521 (30.7, 16.5) -> (34.4528, 23)
  line L522 (34.4528, 23) -> (41.9583, 23)
  line L523 (41.9583, 23) -> (45.7111, 16.5)
  line L524 (45.7111, 16.5) -> (41.9583, 10)
  line L525 (65.6583, 10) -> (58.1528, 10)
  line L526 (58.1528, 10) -> (54.4, 16.5)
  line L527 (54.4, 16.5) -> (58.1528, 23)
  line L528 (58.1528, 23) -> (65.6583, 23)
  line L529 (65.6583, 23) -> (69.4111, 16.5)
  line L530 (69.4111, 16.5) -> (65.6583, 10)
  line L531 (89.3583, 10) -> (81.8528, 10)
  line L532 (81.8528, 10) -> (78.1, 16.5)
  line L533 (78.1, 16.5) -> (81.8528, 23)
  line L534 (81.8528, 23) -> (89.3583, 23)
  line L535 (89.3583, 23) -> (93.1111, 16.5)
  line L536 (93.1111, 16.5) -> (89.3583, 10)
  line L537 (113.0583, 10) -> (105.5528, 10)
  line L538 (105.5528, 10) -> (101.8, 16.5)
  line L539 (101.8, 16.5) -> (105.5528, 23)
  line L540 (105.5528, 23) -> (113.0583, 23)
  line L541 (113.0583, 23) -> (116.8111, 16.5)
  line L542 (116.8111, 16.5) -> (113.0583, 10)
  line L543 (136.7583, 10) -> (129.2528, 10)
  line L544 (129.2528, 10) -> (125.5, 16.5)
  line L545 (125.5, 16.5) -> (129.2528, 23)
  line L546 (129.2528, 23) -> (136.7583, 23)
  line L547 (136.7583, 23) -> (140.5111, 16.5)
  line L548 (140.5111, 16.5) -> (136.7583, 10)
  line L549 (22.0111, 121.5) -> (22.5885, 120.5) construction
  line L550 (159.8583, 115) -> (152.3528, 115)
  line L551 (152.3528, 115) -> (148.6, 121.5)
  line L552 (148.6, 121.5) -> (152.3528, 128)
  line L553 (152.3528, 128) -> (159.8583, 128)
  line L554 (159.8583, 128) -> (163.6111, 121.5)
  line L555 (163.6111, 121.5) -> (159.8583, 115)
  line L556 (160.4357, 114) -> (164.1885, 120.5)
  line L557 (164.1885, 107.5) -> (160.4357, 114)
  line L558 (171.694, 107.5) -> (164.1885, 107.5)
  line L559 (175.4468, 114) -> (171.694, 107.5)
  line L560 (171.694, 120.5) -> (175.4468, 114)
  line L561 (164.1885, 120.5) -> (171.694, 120.5)
  line L562 (159.8583, 100) -> (152.3528, 100)
  line L563 (152.3528, 100) -> (148.6, 106.5)
  line L564 (148.6, 106.5) -> (152.3528, 113)
  line L565 (152.3528, 113) -> (159.8583, 113)
  line L566 (159.8583, 113) -> (163.6111, 106.5)
  line L567 (163.6111, 106.5) -> (159.8583, 100)
  line L568 (160.4357, 99) -> (164.1885, 105.5)
  line L569 (164.1885, 92.5) -> (160.4357, 99)
  line L570 (171.694, 92.5) -> (164.1885, 92.5)
  line L571 (175.4468, 99) -> (171.694, 92.5)
  line L572 (171.694, 105.5) -> (175.4468, 99)
  line L573 (164.1885, 105.5) -> (171.694, 105.5)
  line L574 (159.8583, 85) -> (152.3528, 85)
  line L575 (152.3528, 85) -> (148.6, 91.5)
  line L576 (148.6, 91.5) -> (152.3528, 98)
  line L577 (152.3528, 98) -> (159.8583, 98)
  line L578 (159.8583, 98) -> (163.6111, 91.5)
  line L579 (163.6111, 91.5) -> (159.8583, 85)
  line L580 (160.4357, 84) -> (164.1885, 90.5)
  line L581 (164.1885, 77.5) -> (160.4357, 84)
  line L582 (171.694, 77.5) -> (164.1885, 77.5)
  line L583 (175.4468, 84) -> (171.694, 77.5)
  line L584 (171.694, 90.5) -> (175.4468, 84)
  line L585 (164.1885, 90.5) -> (171.694, 90.5)
  line L586 (159.8583, 70) -> (152.3528, 70)
  line L587 (152.3528, 70) -> (148.6, 76.5)
  line L588 (148.6, 76.5) -> (152.3528, 83)
  line L589 (152.3528, 83) -> (159.8583, 83)
  line L590 (159.8583, 83) -> (163.6111, 76.5)
  line L591 (163.6111, 76.5) -> (159.8583, 70)
  line L592 (160.4357, 69) -> (164.1885, 75.5)
  line L593 (164.1885, 62.5) -> (160.4357, 69)
  line L594 (171.694, 62.5) -> (164.1885, 62.5)
  line L595 (175.4468, 69) -> (171.694, 62.5)
  line L596 (171.694, 75.5) -> (175.4468, 69)
  line L597 (164.1885, 75.5) -> (171.694, 75.5)
  line L598 (159.8583, 55) -> (152.3528, 55)
  line L599 (152.3528, 55) -> (148.6, 61.5)
  line L600 (148.6, 61.5) -> (152.3528, 68)
  line L601 (152.3528, 68) -> (159.8583, 68)
  line L602 (159.8583, 68) -> (163.6111, 61.5)
  line L603 (163.6111, 61.5) -> (159.8583, 55)
  line L604 (160.4357, 54) -> (164.1885, 60.5)
  line L605 (164.1885, 47.5) -> (160.4357, 54)
  line L606 (171.694, 47.5) -> (164.1885, 47.5)
  line L607 (175.4468, 54) -> (171.694, 47.5)
  line L608 (171.694, 60.5) -> (175.4468, 54)
  line L609 (164.1885, 60.5) -> (171.694, 60.5)
  line L610 (159.8583, 40) -> (152.3528, 40)
  line L611 (152.3528, 40) -> (148.6, 46.5)
  line L612 (148.6, 46.5) -> (152.3528, 53)
  line L613 (152.3528, 53) -> (159.8583, 53)
  line L614 (159.8583, 53) -> (163.6111, 46.5)
  line L615 (163.6111, 46.5) -> (159.8583, 40)
  line L616 (160.4357, 39) -> (164.1885, 45.5)
  line L617 (164.1885, 32.5) -> (160.4357, 39)
  line L618 (171.694, 32.5) -> (164.1885, 32.5)
  line L619 (175.4468, 39) -> (171.694, 32.5)
  line L620 (171.694, 45.5) -> (175.4468, 39)
  line L621 (164.1885, 45.5) -> (171.694, 45.5)
  line L622 (159.8583, 25) -> (152.3528, 25)
  line L623 (152.3528, 25) -> (148.6, 31.5)
  line L624 (148.6, 31.5) -> (152.3528, 38)
  line L625 (152.3528, 38) -> (159.8583, 38)
  line L626 (159.8583, 38) -> (163.6111, 31.5)
  line L627 (163.6111, 31.5) -> (159.8583, 25)
  line L628 (160.4357, 24) -> (164.1885, 30.5)
  line L629 (164.1885, 17.5) -> (160.4357, 24)
  line L630 (171.694, 17.5) -> (164.1885, 17.5)
  line L631 (175.4468, 24) -> (171.694, 17.5)
  line L632 (171.694, 30.5) -> (175.4468, 24)
  line L633 (164.1885, 30.5) -> (171.694, 30.5)
  line L634 (159.8583, 10) -> (152.3528, 10)
  line L635 (152.3528, 10) -> (148.6, 16.5)
  line L636 (148.6, 16.5) -> (152.3528, 23)
  line L637 (152.3528, 23) -> (159.8583, 23)
  line L638 (159.8583, 23) -> (163.6111, 16.5)
  line L639 (163.6111, 16.5) -> (159.8583, 10)
  point P0 (92.196, 0)
  point P1 (14.5056, 121.5)
  point P2 (26.3412, 114)
  point P3 (33.8468, 9)
  point P4 (18.8357, 9)
  point P5 (22.5885, 15.5)
  point P6 (30.094, 15.5)
  point P7 (57.5468, 9)
  point P8 (42.5357, 9)
  point P9 (46.2885, 15.5)
  point P10 (53.794, 15.5)
  point P11 (81.2468, 9)
  point P12 (66.2357, 9)
  point P13 (69.9885, 15.5)
  point P14 (77.494, 15.5)
  point P15 (104.9468, 9)
  point P16 (89.9357, 9)
  point P17 (93.6885, 15.5)
  point P18 (101.194, 15.5)
  point P19 (128.6468, 9)
  point P20 (113.6357, 9)
  point P21 (117.3885, 15.5)
  point P22 (124.894, 15.5)
  point P23 (152.3468, 9)
  point P24 (137.3357, 9)
  point P25 (141.0885, 15.5)
  point P26 (148.594, 15.5)
  point P27 (151.7468, 114)
  point P28 (151.7468, 99)
  point P29 (151.7468, 84)
  point P30 (151.7468, 69)
  point P31 (151.7468, 54)
  point P32 (151.7468, 39)
  point P33 (151.7468, 24)
  point P34 (164.1885, 15.5)
  point P35 (171.694, 15.5)
  dimension "d16" = 13
  dimension "d17" = 3
  dimension "d19" = 3
  dimension "d22" = 23.7
  dimension "d25" = 15
  dimension "d47" = 1
  dimension "d51" = 23.1
  dimension "d134" = 2
  dimension "d135" = 1
  dimension "d136" = 1.0248
  constraints: 1274 end point, 5 parallel, 4 horizontal, 4 vertical, 1 collinear, 1 perpendicular, 1295 other
  measures "d16" distance between parallel lines of L12 L9
  measures "d17" distance from line of L6 L10.end
  measures "d19" distance between parallel lines of L7 L12
  measures "d22" distance of L9.start L21.start
  measures "d25" distance of L9.start L81.start
  measures "d47" distance between parallel lines of L85 L17
  measures "d51" distance of L63.start point (151.747, 114)
  measures "d134" distance between parallel lines of L84 L9
  measures "d135" distance between parallel lines of L18 L14
  measures "d136" distance between parallel lines of L20 L22
extrude "HonycombLongSide" cut sketch "LongerHonycomb" against normal blind 140 contours L9 L10 L11 L12 L13 L14 | L15 L16 L17 L18 L19 L20 | L21 L22 L23 L24 L25 L26 | L27 L28 L29 L30 L31 L32 | L33 L34 L35 L36 L37 L38 | L39 L40 L41 L42 L43 L44 | L45 L46 L47 L48 L49 L50 | L51 L52 L53 L54 L55 L56 | L57 L58 L59 L60 L61 L62 | L63 L64 L65 L66 L67 L68 | L69 L70 L71 L72 L73 L74 | L75 L76 L77 L78 L79 L80 | L81 L82 L83 L84 L85 L86 | L87 L88 L89 L90 L91 L92 | L93 L94 L95 L96 L97 L98 | L99 L100 L101 L102 L103 L104 | L105 L106 L107 L108 L109 L110 | L111 L112 L113 L114 L115 L116 | L117 L118 L119 L120 L121 L122 | L123 L124 L125 L126 L127 L128 | L129 L130 L131 L132 L133 L134 | L135 L136 L137 L138 L139 L140 | L141 L142 L143 L144 L145 L146 | L147 L148 L149 L150 L151 L152 | L153 L154 L155 L156 L157 L158 | L159 L160 L161 L162 L163 L164 | L165 L166 L167 L168 L169 L170 | L171 L172 L173 L174 L175 L176 | L177 L178 L179 L180 L181 L182 | L183 L184 L185 L186 L187 L188 | L189 L190 L191 L192 L193 L194 | L195 L196 L197 L198 L199 L200 | L201 L202 L203 L204 L205 L206 | L207 L208 L209 L210 L211 L212 | L213 L214 L215 L216 L217 L218 | L219 L220 L221 L222 L223 L224 | L225 L226 L227 L228 L229 L230 | L231 L232 L233 L234 L235 L236 | L237 L238 L239 L240 L241 L242 | L243 L244 L245 L246 L247 L248 | L249 L250 L251 L252 L253 L254 | L255 L256 L257 L258 L259 L260 | L261 L262 L263 L264 L265 L266 | L267 L268 L269 L270 L271 L272 | L273 L274 L275 L276 L277 L278 | L279 L280 L281 L282 L283 L284 | L285 L286 L287 L288 L289 L290 | L291 L292 L293 L294 L295 L296 | L297 L298 L299 L300 L301 L302 | L303 L304 L305 L306 L307 L308 | L309 L310 L311 L312 L313 L314 | L315 L316 L317 L318 L319 L320 | L321 L322 L323 L324 L325 L326 | L327 L328 L329 L330 L331 L332 | L333 L334 L335 L336 L337 L338 | L339 L340 L341 L342 L343 L344 | L345 L346 L347 L348 L349 L350 | L351 L352 L353 L354 L355 L356 | L357 L358 L359 L360 L361 L362 | L363 L364 L365 L366 L367 L368 | L369 L370 L371 L372 L373 L374 | L375 L376 L377 L378 L379 L380 | L381 L382 L383 L384 L385 L386 | L387 L388 L389 L390 L391 L392 | L393 L394 L395 L396 L397 L398 | L399 L400 L401 L402 L403 L404 | L405 L406 L407 L408 L409 L410 | L411 L412 L413 L414 L415 L416 | L417 L418 L419 L420 L421 L422 | L423 L424 L425 L426 L427 L428 | L429 L430 L431 L432 L433 L434 | L435 L436 L437 L438 L439 L440 | L441 L442 L443 L444 L445 L446 | L447 L448 L449 L450 L451 L452 | L453 L454 L455 L456 L457 L458 | L459 L460 L461 L462 L463 L464 | L465 L466 L467 L468 L469 L470 | L471 L472 L473 L474 L475 L476 | L477 L478 L479 L480 L481 L482 | L483 L484 L485 L486 L487 L488 | L489 L490 L491 L492 L493 L494 | L495 L496 L497 L498 L499 L500 | L501 L502 L503 L504 L505 L506 | L507 L508 L509 L510 L511 L512 | L513 L514 L515 L516 L517 L518 | L519 L520 L521 L522 L523 L524 | L525 L526 L527 L528 L529 L530 | L531 L532 L533 L534 L535 L536 | L537 L538 L539 L540 L541 L542 | L543 L544 L545 L546 L547 L548 | L550 L551 L552 L553 L554 L555 | L556 L561 L560 L559 L558 L557 | L562 L563 L564 L565 L566 L567 | L568 L573 L572 L571 L570 L569 | L574 L575 L576 L577 L578 L579 | L580 L585 L584 L583 L582 L581 | L586 L587 L588 L589 L590 L591 | L592 L597 L596 L595 L594 L593 | L598 L599 L600 L601 L602 L603 | L604 L609 L608 L607 L606 L605 | L610 L611 L612 L613 L614 L615 | L616 L621 L620 L619 L618 L617 | L622 L623 L624 L625 L626 L627 | L628 L633 L632 L631 L630 L629 | L634 L635 L636 L637 L638 L639